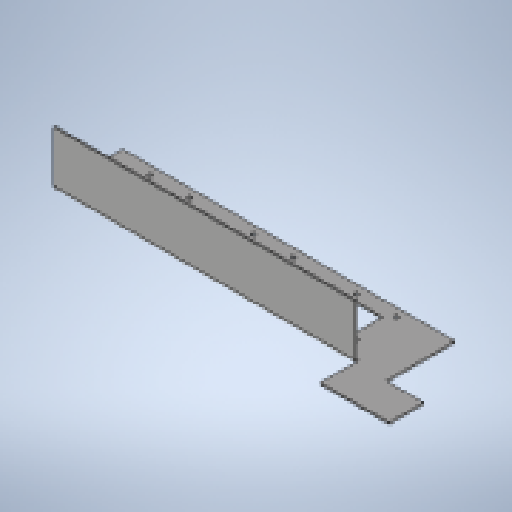
# Autodesk Inventor part: PRS-1423 BOTTOM FDS diameter way down_CPY
Saved by Autodesk Inventor 2026.2 (Build 302298010, 298A)
## iProperties
Created: 2024-12-09
Part Number: PRS-1423 BOTTOM FDS diameter way down_CPY
Material: Stainless Steel
Document SubType Name: Sheet Metal
Designer: admin
Mass: 794.317 g
Surface Area: 1024.01 cm^2
Volume: 99.2896 cm^3
Density: 8 g/cm^3
Flat Pattern Width: 14.0202 cm
Flat Pattern Length: 43 cm
Flat Pattern Area: 602.869 cm^2
Sheet Metal Rule: AISI304 2mm Die16
Sheet Metal Width: 140,202 mm
Sheet Metal Length: 430,000 mm
Sheet Metal Area: 60286,856 mm^2
Appearance: Default
d86: 30,000 mm
d87: 30,000 mm
d93: 30,000 mm
d94: 30,000 mm
Author: user
Autodesk Inventor part; units mm, degrees
ref_plane "YZ Plane" through (0, 0, 0) normal (1, 0, 0) x (0, 1, 0)
ref_plane "XZ Plane" through (0, 0, 0) normal (0, 1, 0) x (-1, 0, 0)
ref_plane "XY Plane" through (0, 0, 0) normal (0, 0, 1) x (1, 0, 0)
sketch "Sketch12" plane through (0, 0, 0) normal (0, 0, -1) x (-1, 0, 0)
  line L0 (0, 0) -> (-80, 0)
  line L1 (-80, 0) -> (-80, -120)
  line L2 (-80, -120) -> (0, -120)
  line L3 (0, -120) -> (0, 0)
  line L4 (-80, 0) -> (-36.3011, 0)
  line L5 (-36.3011, 0) -> (-36.3011, -79.996)
  line L6 (-36.3011, -79.996) -> (-80, -79.996)
  line L7 (-80, -79.996) -> (-80, 0)
  point P0 (-36.3011, 0)
  point P1 (-80, -79.996)
  dimension "d107" = 80
  dimension "d108" = 120
  measures "d107" distance of L2.end L1.end
  measures "d108" distance of L1.end L0.end
sketch "Sketch1" plane through (0, 0, 0) normal (0, 0, 1) x (1, 0, 0)
  line L0 (0, 0) -> (-350, 0)
  line L1 (0, -80) -> (0, 0)
  line L2 (-350, 0) -> (-350, -80)
  line L3 (-350, -80) -> (0, -80)
  point P0 (0, -40)
  dimension "d32" = 80
  dimension "d60" = 80
  dimension "d61" = 350
  measures "d32" distance of L1.start L0.start
  measures "d60" distance of L0.end L2.end
  measures "d61" distance between parallel lines of L1 L2
extrude "Plate1" add sketch "Sketch1" along normal blind 2
sketch "Sketch11" plane through (0, 0, 0) normal (0, 0, -1) x (-1, 0, 0)
  line L0 (60.25, -48.25) -> (29.75, -48.25)
  line L1 (29.75, -48.25) -> (29.75, -17.75)
  line L2 (29.75, -17.75) -> (60.25, -17.75)
  line L3 (60.25, -17.75) -> (60.25, -48.25)
  line L4 (60.25, -48.25) -> (29.75, -17.75) construction
  line L5 (29.75, -48.25) -> (60.25, -17.75) construction
  circle A0 centre (68, -56) radius 2.5
  circle A1 centre (22, -56) radius 2.5
  circle A2 centre (22, -10) radius 2.5
  circle A3 centre (68, -10) radius 2.5
  line L6 (29.75, -48.25) -> (22, -56) construction
  line L7 (0, -80) -> (0, 0) projected
  line L8 (0, 0) -> (350, 0) projected
  line L9 (350, -80) -> (0, -80) projected
  line L10 (22, -10) -> (68, -10) construction
  line L11 (68, -10) -> (68, -56) construction
  line L12 (68, -56) -> (22, -56) construction
  line L13 (22, -56) -> (22, -10) construction
  point P0 (45, -33)
  dimension "d88" = 30.5
  dimension "d89" = 30.5
  dimension "d90" = 5
  dimension "d92" = 10.9602
  dimension "d95" = 45
  dimension "d105" = 46
  dimension "d106" = 10
  constraints: 22 end point, 4 centre point, 4 parallel, 4 point on line, 3 equal radius, 2 horizontal, 2 midpoint, 2 perpendicular
  measures "d88" distance of L0.start L6.start
  measures "d89" distance of L6.start L1.end
  measures "d90" diameter of A0
  measures "d92" distance of L6.end L6.start
  measures "d95" distance from line of point (45, -33) L7
  measures "d105" distance of L10.end L11.end
  measures "d106" distance between parallel lines of L10 L8
extrude "Extrusion2" cut sketch "Sketch11" against normal through all
sketch "Sketch9" plane through (-350, -78, 0) normal (0, -1, 0) x (1, 0, 0)
  line L0 (350, 0) -> (0, 0)
  line L1 (0, 0) -> (0, -64)
  line L2 (0, -64) -> (350, -64)
  line L3 (350, -64) -> (350, 0)
  constraints: 6 end point, 1 horizontal, 1 perpendicular, 1 vertical
edge flange "Flange3" height 64 angle 90 thickness 2 bend radius 2.75 thickness toward (0, -1, 0) relief round relief width 2 relief depth 1 edges at (-175, -80, 0) wall of the first edge with corners at (0, -78, 0) (-350, -78, 0) (-350, -78, 64) (0, -78, 64)
bend "Bend3"
corner "Corner3"
pattern_linear "Rectangular Pattern2" count 3 spacing 120 along (-1, 0, 0) of "Extrusion2"
sheet face with bend "Face3" sketch "Sketch12" thickness 2 toward (0, 0, 1) bend radius 2.75 contours L3 L2 L1 L6 L5 L0
bend "Bend5"
equation "\"d2\" = Thickness"
equation "\"d62\" = BendReliefWidth"
equation "\"d63\" = BendReliefDepth"
equation "\"d64\" = MinimumRemnant"
equation "\"d65\" = TransitionRadius"
equation "\"d66\" = MAIN_7_central_window_width + 2 * Thickness"
equation "\"d68\" = BendRadius"
equation "\"d69\" = CornerReliefSize"
equation "\"d70\" = GapSize"
equation "\"d71\" = JacobiRadiusSize"
equation "\"BendReliefWidth\" = Thickness"
equation "\"BendReliefDepth\" = 0.5 * Thickness"
equation "\"CornerReliefSize\" = 4 * Thickness"
equation "\"MinimumRemnant\" = 2 * Thickness"
equation "\"TransitionRadius\" = BendRadius"
equation "\"JacobiRadiusSize\" = BendRadius"
equation "\"GapSize\" = Thickness"
equation "\"Thickness\" = 2"
equation "\"MAIN_7_central_window_width\" = 60"
equation "\"BendRadius\" = 2.75"
body "Solid1"
